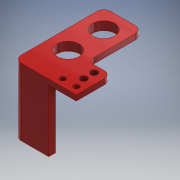
# Autodesk Inventor part: UltrasonicBase
Saved by Autodesk Inventor 2018.3 (Build 223284000, 284)
## iProperties
Created: 2020-03-24
Part Number: UltrasonicBase
Material: Generic
Document SubType Name: Modeling
Designer: Ivan
Density: 1 g/cm^3
Appearance: Default
Author: Ivan
Autodesk Inventor part; units mm, degrees
ref_plane "YZ Plane" through (0, 0, 0) normal (1, 0, 0) x (0, 1, 0)
ref_plane "XZ Plane" through (0, 0, 0) normal (0, 1, 0) x (-1, 0, 0)
ref_plane "XY Plane" through (0, 0, 0) normal (0, 0, 1) x (1, 0, 0)
sketch "Sketch1" plane through (0, 0, 0) normal (0, 0, 1) x (1, 0, 0)
  line L0 (0, 0) -> (-45, 0)
  line L1 (-45, 0) -> (-45, 65)
  line L2 (-45, 65) -> (0, 65)
  line L3 (0, 65) -> (0, 0)
  dimension "d0" = 45
  dimension "d1" = 65
  constraints: 8 end point, 2 parallel, 1 horizontal, 1 perpendicular
  measures "d0" distance between parallel lines of L3 L1
  measures "d1" distance between parallel lines of L0 L2
extrude "Extrusion1" add sketch "Sketch1" along normal blind 4
sketch "Sketch2" plane through (0, 0, 4) normal (0, 0, 1) x (1, 0, 0)
  circle A0 centre (-31, 51) radius 8
  circle A1 centre (-31, 25.117) radius 8
  line L0 (-45, 65) -> (-45, 0) projected
  line L1 (0, 65) -> (-45, 65) projected
  point P0 (0, 0)
  dimension "d4" = 16
  dimension "d5" = 16
  dimension "d6" = 14
  dimension "d7" = 14
  dimension "d8" = 25.883
  constraints: 2 centre point, 1 vertical alignment
  measures "d4" diameter of A0
  measures "d5" diameter of A1
  measures "d6" distance from line of L0 A0.centre
  measures "d7" distance from line of L1 A0.centre
  measures "d8" distance of A1.centre A0.centre
fillet "Fillet3" radius 5 1 edges at (-45, 0, 2)
sketch "Sketch4" plane through (0, 0, 4) normal (0, 0, 1) x (1, 0, 0)
  circle A0 centre (-5, 5.2) radius 2
  line L0 (0, 0) -> (0, 65) projected
  line L1 (-40, 0) -> (0, 0) projected
  circle A1 centre (-15, 5.2) radius 2
  point P0 (0, 60)
  dimension "d20" = 4
  dimension "d21" = 5
  dimension "d22" = 5.2
  dimension "d24" = 10
  dimension "d27" = 4
  constraints: 2 centre point, 1 horizontal alignment
  measures "d20" diameter of A0
  measures "d21" distance from line of L0 A0.centre
  measures "d22" distance from line of L1 A0.centre
  measures "d24" distance of A0.centre A1.centre
  measures "d27" diameter of A1
extrude "Extrusion5" cut sketch "Sketch4" against normal through all
sketch "Sketch6" plane through (0, 0, 0) normal (0, 0, -1) x (-1, 0, 0)
  circle A0 centre (31, 25.117) radius 8 projected
  circle A1 centre (31, 51) radius 8 projected
  circle A2 centre (31, 51) radius 11
  circle A3 centre (31, 25.117) radius 11
  point P0 (0, 0)
  dimension "d34" = 22
  dimension "d35" = 22
  constraints: 2 centre point, 2 coincident
  measures "d34" diameter of A2
  measures "d35" diameter of A3
extrude "Extrusion8" add sketch "Sketch6" along normal blind 3
fillet "Fillet4" radius 1 4 edges at (-20, 51, -3) (-23, 51, -3) (-20, 25.117, -3) (-23, 25.117, -3)
extrude "Extrusion9" cut sketch "Sketch2" against normal through all
sketch "Sketch7" plane through (0, 0, 4) normal (0, 0, 1) x (1, 0, 0)
  line L0 (-17, 65) -> (0, 65)
  line L1 (0, 65) -> (0, 25.4)
  line L2 (0, 25.4) -> (-17, 25.4)
  line L3 (-17, 25.4) -> (-17, 65)
  circle A0 centre (-5, 5.2) radius 2 projected
  line L4 (0, 0) -> (0, 65) projected
  circle A1 centre (-31, 25.117) radius 8 projected
  line L5 (0, 65) -> (-45, 65) projected
  point P0 (0, 60)
  point P1 (-5, 65)
  point P2 (-35, 65)
  dimension "d41" = 20.2
  dimension "d42" = 14
  constraints: 8 end point, 2 collinear, 2 parallel, 1 horizontal, 1 perpendicular
  measures "d41" distance from line of A0.centre L2
  measures "d42" distance from line of L3 A1.centre
extrude "Extrusion10" cut sketch "Sketch7" against normal through all contours L0 L1 L2 L3
fillet "Fillet6" radius 5 4 edges at (0, 25.4, 2) (-17, 25.4, 2) (-17, 65, 2) (-45, 65, 2)
sketch "Sketch8" plane through (0, 0, 4) normal (0, 0, 1) x (1, 0, 0)
  circle A0 centre (-7.5, 20.4) radius 2.5
  line L0 (0, 0) -> (0, 20.4) projected
  line L1 (-5, 25.4) -> (-12, 25.4) projected
  circle A1 centre (-7.5, 12.9) radius 2.5
  dimension "d47" = 5
  dimension "d48" = 7.5
  dimension "d49" = 5
  dimension "d50" = 5
  dimension "d51" = 7.5
  constraints: 2 centre point, 1 vertical alignment
  measures "d47" diameter of A0
  measures "d48" distance from line of L0 A0.centre
  measures "d49" distance from line of L1 A0.centre
  measures "d50" diameter of A1
  measures "d51" distance of A0.centre A1.centre
extrude "Extrusion11" cut sketch "Sketch8" against normal through all
sketch "Sketch9" plane through (0, 0, 0) normal (0, 0, -1) x (-1, 0, 0)
  arc A0 (40, 0) -> (45, 5) centre (40, 5) ccw projected
  arc A1 (40, 0) -> (44.5826, 3) centre (40, 5) ccw
  line L0 (0, 0) -> (40, 0) projected
  line L1 (40, 0) -> (20, 0)
  line L2 (20, 0) -> (20, 3)
  line L3 (20, 3) -> (40, 3)
  line L4 (40, 3) -> (44.5826, 3)
  dimension "d54" = 20
  dimension "d55" = 3
  constraints: 8 end point, 2 horizontal, 2 point on circle, 1 centre point, 1 coincident, 1 parallel, 1 perpendicular, 1 point on line, 1 vertical alignment
  measures "d54" distance of L2.end L3.end
  measures "d55" distance of L1.end L2.end
extrude "Extrusion12" add sketch "Sketch9" along normal blind 45
sketch "Sketch10" plane through (-44.5826, 3, 0) normal (0, 1, 0) x (1, 0, 0)
  line L0 (24.5826, 0) -> (24.5826, 45) projected
  line L1 (20.4076, 8) -> (19.4076, 8)
  line L2 (19.4076, 8) -> (19.4076, 38)
  line L3 (19.4076, 38) -> (20.4076, 38)
  line L4 (20.4076, 38) -> (20.4076, 8)
  line L5 (4.5826, 45) -> (0, 45) construction
  line L6 (24.5826, 45) -> (0, 45) construction
  line L7 (0, 45) -> (12.2915, 45) construction
  line L8 (24.5826, 45) -> (4.5826, 45) construction
  line L9 (12.2915, 45) -> (12.2915, 35) construction
  line L10 (4.1754, 8) -> (5.1754, 8)
  line L11 (5.1754, 8) -> (5.1754, 38)
  line L12 (5.1754, 38) -> (4.1754, 38)
  line L13 (4.1754, 38) -> (4.1754, 8)
  line L14 (19.7913, 39) -> (4.7913, 39)
  line L15 (4.7913, 39) -> (4.7913, 40)
  line L16 (4.7913, 40) -> (19.7913, 40)
  line L17 (19.7913, 40) -> (19.7913, 39)
  point P0 (44.5826, 0)
  point P1 (12.2913, 39)
  point P2 (12.2913, 45)
  dimension "d62" = 1
  dimension "d63" = 30
  dimension "d65" = 4.175
  dimension "d66" = 12.2915
  dimension "d67" = 10
  dimension "d68" = 90
  dimension "d71" = 7
  dimension "d72" = 15
  dimension "d73" = 1
  dimension "d74" = 1
  constraints: 30 end point, 4 parallel, 4 symmetric about line, 3 horizontal, 3 perpendicular, 2 midpoint, 1 point on line, 1 vertical alignment
  measures "d62" distance of L2.end L3.end
  measures "d63" distance of L1.end L2.end
  measures "d65" distance between parallel lines of L0 L4
  measures "d66" distance of L5.end L7.end
  measures "d67" distance of L7.end L9.end
  measures "d68" angle of L7 L9
  measures "d71" distance between parallel lines of L8 L3
  measures "d72" distance of L15.end L16.end
  measures "d73" distance of L14.end L15.end
  measures "d74" distance between parallel lines of L14 L3
extrude "Extrusion14" cut sketch "Sketch10" against normal blind 1
sketch "Sketch11" plane through (-44.5826, 3, 0) normal (0, 1, 0) x (1, 0, 0)
  line L0 (0, 0) -> (0, 45) projected
  line L1 (24.5826, 0) -> (24.5826, 45) projected
  line L2 (0, 0) -> (24.5826, 0)
  line L3 (24.5826, 0) -> (24.5826, 7.5)
  line L4 (24.5826, 7.5) -> (0, 7.5)
  line L5 (0, 7.5) -> (0, 0)
  point P0 (44.5826, 0)
  dimension "d77" = 7.5
  constraints: 8 end point, 2 parallel, 1 horizontal, 1 perpendicular, 1 point on line
  measures "d77" distance of L3.end L2.end
extrude "Extrusion15" add sketch "Sketch11" along normal blind 2
sketch "Sketch12" plane through (-44.5826, 3, -45) normal (0, 1, 0) x (1, 0, 0)
  line L0 (24.5826, -37.5) -> (24.5826, 0) projected
  line L1 (0, -37.5) -> (0, 0) projected
  line L2 (24.5826, 0) -> (0, 0)
  line L3 (0, 0) -> (0, -2.5)
  line L4 (0, -2.5) -> (24.5826, -2.5)
  line L5 (24.5826, -2.5) -> (24.5826, 0)
  line L6 (24.5826, -2.5) -> (21.5826, -2.5)
  line L7 (21.5826, -2.5) -> (21.5826, -37.5)
  line L8 (21.5826, -37.5) -> (24.5826, -37.5)
  line L9 (24.5826, -37.5) -> (24.5826, -2.5)
  line L10 (0, -2.5) -> (3, -2.5)
  line L11 (3, -2.5) -> (3, -37.5)
  line L12 (3, -37.5) -> (0, -37.5)
  line L13 (0, -37.5) -> (0, -2.5)
  point P0 (44.5826, -45)
  dimension "d80" = 2.5
  dimension "d81" = 3
  dimension "d82" = 3
  constraints: 24 end point, 6 parallel, 3 horizontal, 3 perpendicular, 1 point on line
  measures "d80" distance of L3.end L2.end
  measures "d81" distance between parallel lines of L7 L0
  measures "d82" distance between parallel lines of L1 L11
extrude "Extrusion16" add sketch "Sketch12" along normal blind 2
chamfer "Chamfer1" distance 2 angle 45 1 edges at (-32.2913, 3, -42.5)
equation "\"d5\" = d4"
equation "\"d27\" = d20"
equation "\"d48\" = 1.5 * d47"
equation "\"d50\" = d47"
equation "\"d51\" = 1.5 * d47"
equation "\"d82\" = d81"
body "Solid1"
